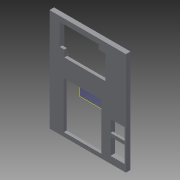
# Autodesk Inventor part: DisplayBottom2
Saved by Autodesk Inventor 2014 SP1 (Build 180222100, 222)
## iProperties
Created: 2014-03-24
Part Number: DisplayBottom2
Material: Generic
Document SubType Name: Modeling
Designer: patrigg
Density: 1 g/cm^3
Appearance: Default
Author: patrigg
Autodesk Inventor part; units mm, degrees
ref_plane "YZ Plane" through (0, 0, 0) normal (1, 0, 0) x (0, 1, 0)
ref_plane "XZ Plane" through (0, 0, 0) normal (0, 1, 0) x (-1, 0, 0)
ref_plane "XY Plane" through (0, 0, 0) normal (0, 0, 1) x (1, 0, 0)
sketch "Sketch2" plane through (0, 0, 0) normal (0, 1, 0) x (-1, 0, 0)
  line L0 (-33.5, -45) -> (33.5, -45)
  line L1 (33.5, -45) -> (33.5, 45)
  line L2 (33.5, 45) -> (-33.5, 45)
  line L3 (-33.5, 45) -> (-33.5, -45)
  line L4 (-33.5, -45) -> (33.5, 45) construction
  line L5 (33.5, -45) -> (-33.5, 45) construction
  point P0 (0, 0)
  dimension "d0" = 67
  dimension "d1" = 90
  constraints: 12 end point, 2 midpoint, 2 parallel, 1 horizontal, 1 perpendicular
  measures "d0" distance of L2.end L1.end
  measures "d1" distance of L1.end L0.end
extrude "Extrusion1" add sketch "Sketch2" along normal blind 4
sketch "Sketch3" plane through (0, 4, 0) normal (0, 1, 0) x (1, 0, 0)
  line L0 (33.5, 45) -> (-33.5, 45) projected
  line L1 (-23.5, -9.5) -> (14.5, -9.5)
  line L2 (14.5, -9.5) -> (14.5, 43)
  line L3 (14.5, 43) -> (-23.5, 43)
  line L4 (-23.5, 43) -> (-23.5, -9.5)
  line L5 (-23.5, -9.5) -> (14.5, 43) construction
  line L6 (14.5, -9.5) -> (-23.5, 43) construction
  line L7 (-33.5, 45) -> (-33.5, -45) projected
  point P0 (0, 0)
  point P1 (-4.5, 16.75)
  dimension "d4" = 38
  dimension "d5" = 52.5
  dimension "d6" = 2
  dimension "d111" = 10
  constraints: 12 end point, 2 midpoint, 2 parallel, 1 horizontal, 1 perpendicular
  measures "d4" distance of L3.end L2.end
  measures "d5" distance of L2.end L1.end
  measures "d6" distance between parallel lines of L0 L3
  measures "d111" distance between parallel lines of L4 L7
extrude "Extrusion2" cut sketch "Sketch3" against normal blind 1.5
sketch "Sketch4" plane through (0, 2.5, 0) normal (0, 1, 0) x (1, 0, 0)
  line L0 (14.5, -9.5) -> (-23.5, -9.5) projected
  line L1 (14.5, 43) -> (14.5, -9.5) projected
  line L2 (-23.5, 43) -> (14.5, 43) projected
  line L3 (-23.5, -9.5) -> (-23.5, 43) projected
  line L4 (-21, 41.5) -> (12, 41.5)
  line L5 (12, 41.5) -> (12, 0.5)
  line L6 (12, 0.5) -> (-21, 0.5)
  line L7 (-21, 0.5) -> (-21, 41.5)
  line L8 (-21, 41.5) -> (12, 0.5) construction
  line L9 (12, 41.5) -> (-21, 0.5) construction
  point P0 (0, 0)
  point P1 (-4.5, 21)
  dimension "d9" = 10
  dimension "d10" = 1.5
  dimension "d11" = 2.5
  dimension "d12" = 2.5
  constraints: 12 end point, 2 midpoint, 2 parallel, 1 horizontal, 1 perpendicular
  measures "d9" distance between parallel lines of L0 L6
  measures "d10" distance between parallel lines of L2 L4
  measures "d11" distance between parallel lines of L1 L5
  measures "d12" distance between parallel lines of L3 L7
extrude "Extrusion3" cut sketch "Sketch4" against normal blind 2.5 contours L4 L5 L6 L7
sketch "Sketch12" plane through (0, 4, 0) normal (0, 1, 0) x (1, 0, 0)
  line L0 (-33.5, -45) -> (33.5, -45) projected
  line L1 (-24.5, -40.5) -> (15.5, -40.5)
  line L2 (15.5, -40.5) -> (15.5, -15.5)
  line L3 (15.5, -15.5) -> (-24.5, -15.5)
  line L4 (-24.5, -15.5) -> (-24.5, -40.5)
  line L5 (-24.5, -40.5) -> (15.5, -15.5) construction
  line L6 (15.5, -40.5) -> (-24.5, -15.5) construction
  line L7 (-23.5, -9.5) -> (-23.5, 43) projected
  point P0 (0, 0)
  point P1 (-4.5, -28)
  point P2 (-4.5, -28)
  point P3 (0, -45)
  dimension "d58" = 40
  dimension "d59" = 25
  dimension "d112" = 1
  constraints: 12 end point, 4 midpoint, 2 parallel, 1 horizontal, 1 perpendicular
  measures "d58" distance of L3.end L2.end
  measures "d59" distance of L2.end L1.end
  measures "d112" distance between parallel lines of L4 L7
extrude "Extrusion10" cut sketch "Sketch12" against normal blind 4
ref_plane "Work Plane1" through (0, 3.75, 0) normal (0, 1, 0) x (1, 0, 0)
sketch "Sketch18" plane through (15.5, 4, 15.5) normal (-1, 0, 0) x (0, 0, 1)
  line L0 (0, 0) -> (25, 0) projected
  line L1 (25, -4) -> (21, -4)
  line L2 (21, -4) -> (21, -1.8)
  line L3 (21, -1.8) -> (25, -1.8)
  line L4 (25, -1.8) -> (25, -4)
  point P0 (-15.5, -4)
  dimension "d88" = 4
  dimension "d89" = 1.8
  constraints: 8 end point, 2 parallel, 1 horizontal, 1 perpendicular
  measures "d88" distance of L2.end L3.end
  measures "d89" distance between parallel lines of L3 L0
extrude "Extrusion17" add sketch "Sketch18" along normal blind 6
sketch "Sketch20" plane through (-24.5, 4, 40.5) normal (1, 0, 0) x (0, 0, -1)
  line L0 (0, 0) -> (25, 0) projected
  line L1 (25, -4) -> (19, -4)
  line L2 (19, -4) -> (19, -1.8)
  line L3 (19, -1.8) -> (25, -1.8)
  line L4 (25, -1.8) -> (25, -4)
  point P0 (40.5, -4)
  dimension "d96" = 6
  dimension "d97" = 1.8
  constraints: 8 end point, 2 parallel, 1 horizontal, 1 perpendicular
  measures "d96" distance of L2.end L3.end
  measures "d97" distance between parallel lines of L3 L0
extrude "Extrusion19" add sketch "Sketch20" along normal blind 4
sketch "Sketch22" plane through (0, 0, 0) normal (0, -1, 0) x (1, 0, 0)
  line L0 (33.5, 45) -> (33.5, -45) projected
  line L1 (-33.5, 45) -> (33.5, 45) projected
  line L2 (32.5, -39) -> (20, -39)
  line L3 (20, -39) -> (20, -11)
  line L4 (20, -11) -> (32.5, -11)
  line L5 (32.5, -11) -> (32.5, -39)
  point P0 (0, 0)
  dimension "d102" = 1
  dimension "d103" = 12.5
  dimension "d107" = 84
  dimension "d110" = 28
  constraints: 8 end point, 2 parallel, 1 horizontal, 1 perpendicular
  measures "d102" distance between parallel lines of L5 L0
  measures "d103" distance between parallel lines of L3 L5
  measures "d107" distance between parallel lines of L2 L1
  measures "d110" distance between parallel lines of L4 L2
extrude "Extrusion21" cut sketch "Sketch22" against normal up to next
sketch "Sketch23" plane through (0, 4, 0) normal (0, 1, 0) x (1, 0, 0)
  line L0 (-24.5, -15.5) -> (15.5, -15.5) projected
  line L1 (14.5, 43) -> (14.5, -9.5) projected
  line L2 (14.5, -9.5) -> (-23.5, -9.5) projected
  line L3 (-23.5, -9.5) -> (-23.5, 43) projected
  line L4 (-21.5, -9.5) -> (-21.5, -15.5)
  line L5 (12.5, -9.5) -> (12.5, -15.5)
  point P0 (0, 0)
  dimension "d114" = 2
  dimension "d115" = 2
  constraints: 4 end point, 4 point on line, 2 perpendicular
  measures "d114" distance between parallel lines of L4 L3
  measures "d115" distance between parallel lines of L1 L5
extrude "Extrusion22" cut sketch "Sketch23" against normal up to surface (1.5 mm away)
sketch "Sketch24" plane through (32.5, 0, -39) normal (-1, 0, 0) x (0, 0, 1)
  line L0 (0, 0) -> (0, 4) projected
  line L1 (28, 0) -> (0, 0) projected
  line L2 (14.5, 0) -> (17.5, 0)
  line L3 (17.5, 0) -> (17.5, 2)
  line L4 (17.5, 2) -> (14.5, 2)
  line L5 (14.5, 2) -> (14.5, 0)
  line L6 (14.5, 0) -> (17.5, 2) construction
  line L7 (17.5, 0) -> (14.5, 2) construction
  point P0 (16, 1)
  dimension "d118" = 3
  dimension "d119" = 2
  dimension "d120" = 16
  constraints: 12 end point, 2 midpoint, 2 parallel, 1 collinear, 1 horizontal, 1 perpendicular
  measures "d118" distance of L4.end L3.end
  measures "d119" distance of L3.end L2.end
  measures "d120" distance from line of L0 point (16, 1)
extrude "Extrusion23" add sketch "Sketch24" along normal up to next
sketch "Sketch25" plane through (32.5, 2, -21.5) normal (0, 1, 0) x (1, 0, 0)
  line L0 (0, 0) -> (-12.5, 0) projected
  line L1 (0, 3) -> (-12.5, 3) projected
  line L2 (-7.75, 1) -> (-4.75, 1)
  line L3 (-4.75, 1) -> (-4.75, 3)
  line L4 (-4.75, 3) -> (-7.75, 3)
  line L5 (-7.75, 3) -> (-7.75, 1)
  line L6 (-7.75, 1) -> (-4.75, 3) construction
  line L7 (-4.75, 1) -> (-7.75, 3) construction
  point P0 (-32.5, -21.5)
  point P1 (-6.25, 2)
  point P2 (-6.25, 2)
  point P3 (-6.25, 0)
  dimension "d123" = 3
  dimension "d124" = 2
  constraints: 12 end point, 4 midpoint, 2 parallel, 1 collinear, 1 horizontal, 1 perpendicular, 1 vertical alignment
  measures "d123" distance of L4.end L3.end
  measures "d124" distance of L3.end L2.end
extrude "Extrusion24" cut sketch "Sketch25" against normal blind 0.5
fillet "Fillet6" radius 1 1 edges at (26.25, 1.5, -24.5)
sketch "Sketch26" plane through (32.5, 2, -21.5) normal (0, 1, 0) x (1, 0, 0)
  line L0 (0, 0) -> (-12.5, 0) projected
  line L1 (0, 3) -> (0, 0) projected
  circle A0 centre (-10.375, 1.5) radius 1.25
  circle A1 centre (-2.125, 1.5) radius 1.25
  point P0 (-32.5, -21.5)
  point P1 (-6.25, 1.5)
  point P2 (0, 1.5)
  point P3 (-6.25, 0)
  dimension "d128" = 2.5
  dimension "d129" = 2.5
  dimension "d130" = 4.125
  dimension "d131" = 8.25
  constraints: 3 horizontal alignment, 2 centre point, 2 midpoint, 1 vertical alignment
  measures "d128" diameter of A0
  measures "d129" diameter of A1
  measures "d130" distance of point (-6.25, 1.5) A0.centre
  measures "d131" distance of A1.centre A0.centre
extrude "Extrusion25" add sketch "Sketch26" along normal blind 1.5
chamfer "Chamfer3" distance 0.5 angle 45 2 edges at (29.125, 3.5, -23) (20.875, 3.5, -23)
body "Solid1"
